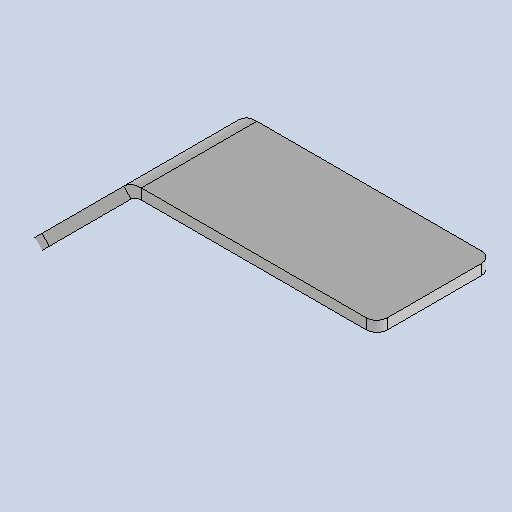
# Autodesk Inventor part: TKS 3563 FDS support cup
Saved by Autodesk Inventor 2025 (Build 290162010, 162A)
## iProperties
Created: 2025-06-24
Part Number: TKS 3563 FDS support cup
Material: Stainless Steel
Document SubType Name: Sheet Metal
Designer: admin
Mass: 14.3451 g
Surface Area: 20.2627 cm^2
Volume: 1.79313 cm^3
Density: 8 g/cm^3
Flat Pattern Width: 2.2 cm
Flat Pattern Length: 7.57444 cm
Flat Pattern Area: 16.6638 cm^2
Sheet Metal Rule: AISI304 2mm Die16
Sheet Metal Width: 22,000 mm
Sheet Metal Length: 75,744 mm
Sheet Metal Area: 1666,377 mm^2
Appearance: Default
Author: user
Autodesk Inventor part; units mm, degrees
ref_plane "YZ Plane" through (0, 0, 0) normal (1, 0, 0) x (0, 1, 0)
ref_plane "XZ Plane" through (0, 0, 0) normal (0, 1, 0) x (-1, 0, 0)
ref_plane "XY Plane" through (0, 0, 0) normal (0, 0, 1) x (1, 0, 0)
sketch "Sketch1" plane through (0, 0, 0) normal (0, 0, 1) x (1, 0, 0)
  line L0 (-22, -11) -> (22, -11)
  line L1 (22, -11) -> (22, 11)
  line L2 (22, 11) -> (-22, 11)
  line L3 (-22, 11) -> (-22, -11)
  line L4 (-22, -11) -> (22, 11) construction
  line L5 (22, -11) -> (-22, 11) construction
  point P0 (0, 0)
  dimension "d154" = 44
  dimension "d155" = 22
  measures "d154" distance of L1.end L2.end
  measures "d155" distance of L0.end L1.end
extrude "Plate5" add sketch "Sketch1" along normal blind 2
fillet "Corner Round1" radius 2 2 edges at (22, 11, 1) (22, -11, 1)
sketch "Sketch10" plane through (-23.4142, 11, 3.4142) normal (0.7071068, 0, -0.7071068) x (0, 1, 0)
  line L0 (-22, 0) -> (0, 0)
  line L1 (0, 0) -> (0, -32)
  line L2 (0, -32) -> (-22, -32)
  line L3 (-22, -32) -> (-22, 0)
  constraints: 8 end point
edge flange "Flange4" height 30 angle 45 thickness 2 bend radius 2.75 thickness toward (0.7071068, 0, -0.7071068) relief round relief width 2 relief depth 1 edges at (-22, 0, 0) wall of the first edge with corners at (-23.4142, -11, 3.4142) (-23.4142, 11, 3.4142) (-46.0416, 11, -19.2132) (-46.0416, -11, -19.2132)
bend "Bend4"
corner "Corner4"
sketch "Sketch11" plane through (-44.6274, -11, -20.6274) normal (0.7071068, 0, -0.7071068) x (-0.7071068, 0, -0.7071068)
  line L0 (-28.0325, 22) -> (-28.0325, 0) construction
  line L1 (0, 0) -> (-28.0325, 0) construction
  line L2 (0, 0) -> (0, 22) construction
  line L3 (0, 22) -> (-28.0325, 22) construction
  circle A0 centre (-10, 11) radius 5.5
  point P0 (-46.1421, 11)
  point P1 (0, 11)
  dimension "d192" = 11
  dimension "d193" = 10
  constraints: 1 centre point, 1 horizontal alignment, 1 midpoint
  measures "d192" diameter of A0
  measures "d193" distance from line of A0.centre L2
extrude "Cut3" cut sketch "Sketch11" against normal blind 2
fillet "Corner Round3" radius 6 2 edges at (-45.3345, 11, -19.9203) (-45.3345, -11, -19.9203)
body "Solid3"
